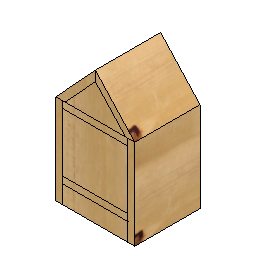
Garduino Housing v12 (Autodesk Fusion 360 design; units mm, degrees)
Autodesk Fusion 360 part; units mm, degrees
sketch "Sketch5" plane through (0, 0, 0) normal (0, 0, 1) x (1, 0, 0)
  line L0 (0, 0) -> (184.15, 0)
  line L1 (184.15, 0) -> (184.15, 19.05)
  line L2 (184.15, 19.05) -> (0, 19.05)
  line L3 (0, 19.05) -> (0, 0)
  line L4 (-46.6311, 0) -> (230.0028, 0) construction
  line L5 (0, -50.8) -> (-19.05, -50.8)
  line L6 (-19.05, -50.8) -> (-19.05, 203.2)
  line L7 (-19.05, 203.2) -> (0, 203.2)
  line L8 (0, 203.2) -> (0, -50.8)
  line L9 (184.15, -50.8) -> (203.2, -50.8)
  line L10 (203.2, -50.8) -> (203.2, 203.2)
  line L11 (203.2, 203.2) -> (184.15, 203.2)
  line L12 (184.15, 203.2) -> (184.15, -50.8)
  line L13 (0, 203.2) -> (184.15, 203.2)
  line L14 (184.15, 203.2) -> (184.15, 184.15)
  line L15 (184.15, 184.15) -> (0, 184.15)
  line L16 (0, 184.15) -> (0, 203.2)
  line L17 (0, 0) -> (184.15, 0)
  line L18 (184.15, 0) -> (184.15, -50.8)
  line L19 (184.15, -50.8) -> (0, -50.8)
  line L20 (0, -50.8) -> (0, 0)
  line L21 (92.075, -50.8) -> (92.075, 323.85) construction
  line L22 (-19.05, 203.2) -> (92.075, 323.85)
  line L23 (203.2, 203.2) -> (92.075, 323.85)
  line L24 (189.1879, 190.2941) -> (92.075, 295.7309)
  line L25 (-5.0379, 190.2941) -> (92.075, 295.7309)
  line L26 (92.075, 295.7309) -> (92.075, 323.85)
  dimension "d72" = 184.15
  dimension "d73" = 19.05
  dimension "d74" = 19.05
  dimension "d75" = 254
  dimension "d76" = 19.05
  dimension "d77" = 50.8
  dimension "d78" = 19.05
  dimension "d79" = 254
  dimension "d80" = 50.8
  dimension "d81" = 184.15
  dimension "d82" = 19.05
  dimension "d83" = 374.65
  dimension "d84" = -19.05
  constraint horizontal L0
  constraint vertical L1
  constraint horizontal L2
  constraint vertical L3
  constraint coincident L0.start L3.end
  constraint perpendicular L3 L4
  constraint horizontal L5
  constraint vertical L6
  constraint horizontal L7
  constraint vertical L8
  constraint coincident L0.start L4
  constraint horizontal L9
  constraint vertical L10
  constraint horizontal L11
  constraint vertical L12
  constraint coincident L0.end L12
  constraint horizontal L13
  constraint vertical L14
  constraint horizontal L15
  constraint vertical L16
  constraint horizontal L17
  constraint vertical L18
  constraint horizontal L19
  constraint vertical L20
  constraint vertical L21
  constraint midpoint L19 L21.start
  measures "d72" distance of L0.start L0.end
  measures "d73" distance of L0.start L2.end
  measures "d74" distance of L5.start L5.end
  measures "d75" distance of L5.start L7.end
  measures "d76" distance of L3 L6
  measures "d77" distance of L4 L5
  measures "d78" distance of L9.start L9.end
  measures "d79" distance of L9.start L11.end
  measures "d80" distance of L4 L9
  measures "d81" distance of L7.end L11.end
  measures "d82" distance of L7.end L15.end
  measures "d83" distance of L21.start L21.end
extrude "Extrude1" add sketch "Sketch5" along normal blind 184.15 contours L3 L5 L6 L7 L8 L16 L20 | L1 L9 L10 L11 L12 L14 L18 makes body 1 at (0, 118.5333, 61.3833) makes body 2 at (184.15, 33.8667, 122.7667)
extrude "Extrude3" add sketch "Sketch5" along normal blind 184.15 separate body contours L0 L1 L2 L3 L8 L12 L17 | L8 L12 L13 L14 L15 L16 L24 L25 | L8 L13 L16 L25 | L12 L13 L14 L24 makes body 3 at (122.7667, 184.15, 61.3833) makes body 4 at (122.7667, 19.05, 61.3833)
extrude "Extrude5" add sketch "Sketch5" along normal blind 19.05 separate body contours L2 L8 L12 L15 makes body 5
extrude "Extrude6" add sketch "Sketch5" against normal blind 19.05 from surface at 184.15 separate body contours L2 L8 L12 L15 makes body 6
extrude "Extrude7" add sketch "Sketch5" along normal blind 184.15 separate body contours L7 L13 L22 L25 L26 makes body 7
extrude "Extrude19" add sketch "Sketch5" along normal blind 184.15 separate body contours L11 L13 L23 L24 L26 makes body 8
extrude "Extrude17" add sketch "Sketch5" along normal blind 19.05 separate body contours L0 L8 L12 L17 L18 L19 L20 makes body 9
extrude "Extrude18" add sketch "Sketch5" against normal blind 19.05 from surface at 184.15 separate body contours L0 L8 L12 L17 L18 L19 L20 makes body 10
extrude "Extrude13" add sketch "Sketch5" along normal blind 19.05 separate body contours L13 L24 L25 makes body 11
extrude "Extrude14" add sketch "Sketch5" against normal blind 19.05 from surface at 184.15 separate body contours L13 L24 L25 makes body 12
sketch "Sketch3" plane through (0, 0, 0) normal (0, -1, 0) x (1, 0, 0)
  line L0 (0, 203.2) -> (0, 0)
  line L1 (44.45, 149.225) -> (171.45, 149.225)
  line L2 (171.45, 149.225) -> (171.45, 34.925)
  line L3 (171.45, 34.925) -> (44.45, 34.925)
  line L4 (44.45, 34.925) -> (44.45, 149.225)
  line L5 (0, 0) -> (184.15, 0)
  line L6 (184.15, 0) -> (184.15, 184.15)
  line L7 (184.15, 184.15) -> (0, 184.15)
  line L8 (0, 184.15) -> (0, 0)
  line L9 (184.15, 0) -> (0, 0)
  line L10 (0, 0) -> (0, 184.15)
  line L11 (0, 184.15) -> (184.15, 184.15)
  line L12 (184.15, 184.15) -> (184.15, 0)
  dimension "d47" = 127
  dimension "d48" = 114.3
  dimension "d89" = 12.7
  dimension "d90" = 34.925
  constraint horizontal L1
  constraint vertical L2
  constraint horizontal L3
  constraint vertical L4
  measures "d47" distance of L1.start L1.end
  measures "d48" distance of L1.start L3.end
  measures "d89" distance of L2 L12
  measures "d90" distance of L1 L7
extrude "Extrude20" cut sketch "Sketch3" against normal up to surface (19.05 mm away) contours L1 L2 L3 L4 bodies 4
ref_plane "WorkPlane2" through (-19.05, 76.2, 92.075) normal (-1, 0, 0) x (0, -1, 0)
sketch "Sketch4" plane through (-19.05, 76.2, 101.6) normal (-1, 0, 0) x (0, 0, -1)
  line L0 (-92.075, 76.2) -> (115.9309, 76.2) construction
  line L1 (111.125, 57.15) -> (-92.075, 57.15) construction
  line L2 (9.525, -127) -> (9.525, 57.15)
  line L3 (111.125, -34.925) -> (-92.075, -34.925)
  line L4 (31.75, -54.61) -> (-12.7, -54.61)
  line L5 (-12.7, -54.61) -> (-12.7, -15.24)
  line L6 (-12.7, -15.24) -> (31.75, -15.24)
  line L7 (31.75, -15.24) -> (31.75, -54.61)
  line L8 (101.6, -127) -> (101.6, 127)
  line L9 (101.6, 127) -> (-101.6, 127)
  line L10 (101.6, -127) -> (101.6, 127)
  line L11 (101.6, 127) -> (-82.55, 127)
  line L12 (-82.55, 127) -> (-82.55, -127)
  line L13 (-82.55, -127) -> (101.6, -127)
  dimension "d54" = 19.05
  dimension "d56" = 44.45
  dimension "d57" = 39.37
  dimension "d58" = 19.685
  dimension "d59" = 22.225
  dimension "d87" = 92.075
  dimension "d88" = 92.075
  constraint midpoint L1 L2.end
  constraint horizontal L4
  constraint vertical L5
  constraint horizontal L6
  constraint vertical L7
  measures "d54" distance of L0 L1
  measures "d56" distance of L4.start L4.end
  measures "d57" distance of L4.start L6.end
  measures "d58" distance of L3 L4
  measures "d59" distance of L2 L7
  measures "d87" distance of L2 L12
  measures "d88" distance of L3 L13
extrude "Extrude16" [suppressed]
